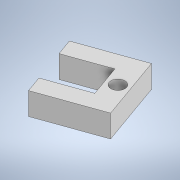
# Autodesk Inventor part: fileholddub
Saved by Autodesk Inventor 2020 (Build 240168000, 168)
## iProperties
Created: 2019-07-05
Part Number: fileholddub
Material: Generic
Document SubType Name: Modeling
Designer: ColinP
Density: 1 g/cm^3
Appearance: Default
Author: ColinP
Autodesk Inventor part; units mm, degrees
ref_plane "YZ Plane" through (0, 0, 0) normal (1, 0, 0) x (0, 1, 0)
ref_plane "XZ Plane" through (0, 0, 0) normal (0, 1, 0) x (-1, 0, 0)
ref_plane "XY Plane" through (0, 0, 0) normal (0, 0, 1) x (1, 0, 0)
sketch "Sketch1" plane through (0, 0, 0) normal (0, 1, 0) x (-1, 0, 0)
  line L0 (6.5094, 9.5985) -> (7.4635, 6.913)
  line L1 (10.1521, -0.6544) -> (11.1062, -3.34)
  line L2 (-11.9694, 3.8348) -> (7.7922, 10.8558)
  line L3 (9.0875, 7.21) -> (-10.6741, 0.1891)
  line L4 (-8.1622, -6.8813) -> (11.5995, 0.1397)
  line L5 (12.8948, -3.5061) -> (-6.8669, -10.5271)
  line L6 (-6.8669, -10.5271) -> (-8.1622, -6.8813)
  line L7 (11.5995, 0.1397) -> (12.8948, -3.5061)
  line L8 (7.7922, 10.8558) -> (9.0875, 7.21)
  line L9 (-10.6741, 0.1891) -> (-11.9694, 3.8348)
  line L10 (6.9865, 8.2558) -> (-11.2395, 1.7804)
  line L11 (10.6292, -1.9972) -> (-7.5968, -8.4726)
  circle A0 centre (-12.8288, -4.5578) radius 1.5875
  line L12 (-12.8288, -4.5578) -> (-11.2395, 1.7804)
  line L13 (-7.5968, -8.4726) -> (-12.8288, -4.5578)
  line L14 (-11.2395, 1.7804) -> (-7.5968, -8.4726)
  line L15 (-6.8669, -10.5271) -> (-11.2395, -12.0806)
  line L16 (-11.2395, -12.0806) -> (-15.6121, 0.2269)
  line L17 (-15.6121, 0.2269) -> (-11.2395, 1.7804)
  line L18 (6.5094, 9.5985) -> (-11.7166, 3.1231)
  line L19 (7.4635, 6.913) -> (-10.7624, 0.4376)
  line L20 (10.1521, -0.6544) -> (-8.0739, -7.1298)
  line L21 (11.1062, -3.34) -> (-7.1197, -9.8154)
  line L22 (11.645, -4.8563) -> (9.3537, 1.5929)
  line L23 (-11.9694, 3.8348) -> (-16.342, 2.2813)
  line L24 (-16.342, 2.2813) -> (-15.6121, 0.2269)
  line L25 (-11.9694, 3.8348) -> (-11.2395, 1.7804)
  line L26 (6.9865, 8.2558) -> (-2.8266, 4.7693)
  line L27 (10.6292, -1.9972) -> (0.8161, -5.4836)
  line L28 (0.8161, -5.4836) -> (1.2932, -6.8264)
  line L29 (0.339, -4.1409) -> (0.8161, -5.4836)
  line L30 (-2.8266, 4.7693) -> (-2.3495, 3.4266)
  line L31 (-2.8266, 4.7693) -> (-3.3037, 6.1121)
  line L32 (-11.9694, 3.8348) -> (-3.5565, 6.8238)
  line L33 (-2.2612, 3.178) -> (-2.3495, 3.4266)
  line L34 (-2.2612, 3.178) -> (-10.6741, 0.1891)
  line L35 (0.339, -4.1409) -> (0.2507, -3.8923)
  line L36 (-8.1622, -6.8813) -> (0.2507, -3.8923)
  line L37 (1.2932, -6.8264) -> (1.546, -7.5381)
  line L38 (-6.8669, -10.5271) -> (1.546, -7.5381)
  line L39 (-6.8669, -10.5271) -> (-7.5968, -8.4726)
  line L40 (-3.3037, 6.1121) -> (-3.5565, 6.8238)
  point P0 (0, 0)
  dimension "d0" = 10.414
  dimension "d1" = 10.414
  constraints: 82 end point, 23 point on line, 12 perpendicular, 5 collinear, 2 midpoint, 1 centre point, 1 parallel
  measures "d0" distance of L10.start L26.end
  measures "d1" distance of L11.start L27.end
extrude "Extrusion1" add sketch "Sketch1" along normal blind 2.54 contours L31 L10 L9 L18 | L18 L9 L2 L40 | L30 L19 L9 L10 | L9 L17 L24 L23 | L33 L3 L9 L19 | L9 L14 L6 L13 A0 L12 | L12 A0 L16 L17 | L12 L13 A0 L16 | A0 L13 L12 | L4 L35 L20 L6 | L13 L6 L15 L16 A0 | L20 L29 L11 L6 | L11 L28 L21 L6 | L21 L37 L5 L6
sketch "Sketch2" plane through (0, 2.54, 0) normal (0, 1, 0) x (1, 0, 0)
  line L0 (11.2395, 12.0806) -> (-1.546, 7.5381) projected
  line L1 (-1.546, 7.5381) -> (2.092, 8.8306)
  line L2 (2.092, 8.8306) -> (3.3873, 5.1848)
  line L3 (-0.2507, 3.8923) -> (8.1622, 6.8813) projected
  line L4 (-0.2507, 3.8923) -> (3.3873, 5.1848)
  line L5 (-1.546, 7.5381) -> (-0.2507, 3.8923) projected
  line L6 (-0.2507, 3.8923) -> (-1.546, 7.5381)
  line L7 (2.2612, -3.178) -> (3.5565, -6.8238) projected
  line L8 (2.2612, -3.178) -> (3.5565, -6.8238)
  line L9 (3.5565, -6.8238) -> (7.1945, -5.5313)
  line L10 (3.5565, -6.8238) -> (16.342, -2.2813) projected
  line L11 (7.1945, -5.5313) -> (5.8992, -1.8855)
  line L12 (10.6741, -0.1891) -> (2.2612, -3.178) projected
  line L13 (2.2612, -3.178) -> (5.8992, -1.8855)
  point P0 (0, 0)
  dimension "d4" = 3.8608
  dimension "d5" = 3.8608
  constraints: 16 end point, 4 point on line, 3 collinear, 3 perpendicular
  measures "d4" distance of L0.end L1.end
  measures "d5" distance of L7.end L9.end
extrude "Extrusion2" add sketch "Sketch2" along normal blind 2.54
sketch "Sketch3" plane through (0, 2.54, 0) normal (0, 1, 0) x (1, 0, 0)
  line L0 (8.1622, 6.8813) -> (10.6741, -0.1891) projected
  line L1 (8.1622, 6.8813) -> (6.8669, 10.5271)
  line L2 (11.2395, 12.0806) -> (-1.546, 7.5381) projected
  line L3 (10.6615, -0.1534) -> (11.9694, -3.8348)
  line L4 (7.1945, -5.5313) -> (16.342, -2.2813) projected
  line L5 (6.8669, 10.5271) -> (2.092, 8.8306)
  line L6 (3.3873, 5.1848) -> (8.1622, 6.8813) projected
  line L7 (3.3873, 5.1848) -> (8.1622, 6.8813)
  line L8 (8.1622, 6.8813) -> (3.3873, 5.1848)
  line L9 (3.3873, 5.1848) -> (2.092, 8.8306) projected
  line L10 (2.092, 8.8306) -> (3.3873, 5.1848)
  line L11 (10.6741, -0.1891) -> (5.8992, -1.8855) projected
  line L12 (5.8992, -1.8855) -> (10.6741, -0.1891)
  line L13 (10.6741, -0.1891) -> (11.9694, -3.8348)
  line L14 (5.8992, -1.8855) -> (7.1945, -5.5313) projected
  line L15 (11.9694, -3.8348) -> (7.1945, -5.5313)
  line L16 (7.1945, -5.5313) -> (5.8992, -1.8855)
  point P0 (0, 0)
  constraints: 20 end point, 5 point on line, 4 collinear, 3 perpendicular
extrude "Extrusion3" add sketch "Sketch3" along normal blind 2.54
sketch "Sketch6" plane through (0, 2.54, 0) normal (0, 1, 0) x (1, 0, 0)
  line L0 (8.1622, 6.8813) -> (10.6741, -0.1891) projected
  line L1 (8.1622, 6.8813) -> (12.5348, 8.4348)
  line L2 (16.342, -2.2813) -> (11.2395, 12.0806) projected
  line L3 (10.6741, -0.1891) -> (15.0468, 1.3644)
  line L4 (15.0468, 1.3644) -> (12.8604, 0.5877)
  line L5 (10.3485, 7.658) -> (12.8604, 0.5877)
  line L6 (10.3485, 7.658) -> (9.0532, 11.3038)
  line L7 (11.2395, 12.0806) -> (-1.546, 7.5381) projected
  line L8 (12.8604, 0.5877) -> (14.1557, -3.0581)
  line L9 (11.9694, -3.8348) -> (16.342, -2.2813) projected
  circle A0 centre (11.6045, 4.1229) radius 1.4859
  point P0 (0, 0)
  dimension "d28" = 2.9718
  constraints: 12 end point, 4 midpoint, 2 point on line, 1 centre point, 1 parallel, 1 perpendicular
  measures "d28" diameter of A0
hole "Hole3" at (11.6045, 2.54, -4.1229) direction (0, -1, 0) diameter 3.175 depth 7.62
sketch "Sketch7" plane through (0, 2.54, 0) normal (0, 1, 0) x (1, 0, 0)
  circle A0 centre (11.6045, 4.1229) radius 1.5875 projected
  line L0 (10.6741, -0.1891) -> (11.9694, -3.8348) projected
  line L1 (11.9694, -3.8348) -> (16.342, -2.2813) projected
  line L2 (16.342, -2.2813) -> (11.2395, 12.0806) projected
  line L3 (11.2395, 12.0806) -> (6.8669, 10.5271) projected
  line L4 (6.8669, 10.5271) -> (8.1622, 6.8813) projected
  line L5 (8.1622, 6.8813) -> (10.6741, -0.1891) projected
  point P0 (0, 0)
extrude "Extrusion4" add sketch "Sketch7" along normal blind 2.54 contours A0 | L5 L4 L3 L2 L1 L0
sketch "Sketch8" plane through (11.6045, 2.54, -4.1229) normal (0, -1, 0) x (1, 0, 0)
  circle A0 centre (0, 0) radius 1.5875 projected
  point P0 (-11.6045, 4.1229)
  constraints: 1 coincident
hole "Hole4" at (11.6045, 2.54, -4.1229) direction (0, 1, 0) diameter 3.175 depth 7.62
sketch "Sketch9" plane through (0, 0, 0) normal (0, -1, 0) x (1, 0, 0)
  line L0 (3.5565, 6.8238) -> (16.342, 2.2813) projected
  line L1 (10.6741, 0.1891) -> (2.2612, 3.178) projected
  line L2 (-0.2507, -3.8923) -> (8.1622, -6.8813) projected
  line L3 (11.2395, -12.0806) -> (-1.546, -7.5381) projected
  line L4 (3.5565, 6.8238) -> (16.342, 2.2813) projected
  line L5 (3.5565, 6.8238) -> (2.9821, 7.0279)
  line L6 (10.5107, 3.6362) -> (3.3304, 6.1873) projected
  line L7 (2.9821, 7.0279) -> (1.6868, 3.3821)
  line L8 (2.2612, 3.178) -> (3.5565, 6.8238) projected
  line L9 (1.6868, 3.3821) -> (2.2612, 3.178)
  line L10 (-1.546, -7.5381) -> (-0.2507, -3.8923) projected
  line L11 (-0.2507, -3.8923) -> (-0.8252, -3.6882)
  line L12 (-0.8252, -3.6882) -> (-2.1204, -7.334)
  line L13 (-2.1204, -7.334) -> (-1.4728, -7.5641)
  point P0 (0, 0)
  dimension "d45" = 0.6096
  constraints: 12 end point, 4 perpendicular, 2 collinear, 1 parallel, 1 point on line
  measures "d45" distance of L0.start L5.end
extrude "Extrusion5" add sketch "Sketch9" against normal blind 5.08
sketch "Sketch12" plane through (2.9821, 0, 7.0279) normal (-0.9422958, 0, 0.3347815) x (0.3347815, 0, 0.9422958)
  line L0 (0, 0) -> (-3.869, 0) projected
  line L1 (0, 0) -> (0, 5.08) projected
  line L2 (-3.869, 5.08) -> (0, 5.08) projected
  line L3 (-3.869, 0) -> (-3.869, 5.08) projected
  line L4 (-11.3724, 0) -> (-15.2414, 0) projected
  line L5 (-11.3724, 0) -> (-11.3724, 5.08) projected
  line L6 (-15.2414, 5.08) -> (-11.3724, 5.08) projected
  line L7 (-15.2414, 0) -> (-15.2414, 5.08) projected
  point P0 (-7.6207, 0)
extrude "Extrusion6" add sketch "Sketch12" along normal blind 0.381
sketch "Sketch15" plane through (2.6231, 0, 7.1554) normal (-0.9422958, 0, 0.3347815) x (0.3347815, 0, 0.9422958)
  line L0 (-11.3724, 5.08) -> (-15.2414, 5.08) projected
  line L1 (-15.2414, 5.08) -> (-15.2414, 0) projected
  point P0 (-7.6207, 0)
  point P1 (-13.3364, 3.175)
  dimension "d93" = 1.905
  dimension "d94" = 1.905
  measures "d93" distance from line of L0 point (-13.336, 3.175)
  measures "d94" distance from line of L1 point (-13.336, 3.175)
hole "Hole10" at (-1.8417, 3.175, -5.4114) direction (0.9422958, 0, -0.3347815) diameter 2.459 depth 8.7884 thread size "M3x0.5" class "6H" standard "ISO Metric profile"
sketch "Sketch16" plane through (2.6231, 0, 7.1554) normal (-0.9422958, 0, 0.3347815) x (0.3347815, 0, 0.9422958)
  line L0 (0, 5.08) -> (-3.869, 5.08) projected
  line L1 (0, 0) -> (0, 5.08) projected
  point P0 (-7.6207, 0)
  point P1 (-1.905, 3.175)
  dimension "d102" = 1.905
  dimension "d103" = 1.905
  measures "d102" distance from line of L0 point (-1.905, 3.175)
  measures "d103" distance from line of L1 point (-1.905, 3.175)
hole "Hole11" at (1.9853, 3.175, 5.3604) direction (0.9422958, 0, -0.3347815) diameter 2.459 depth 8.7884 thread size "M3x0.5" class "6H" standard "ISO Metric profile"
body "Solid1"
